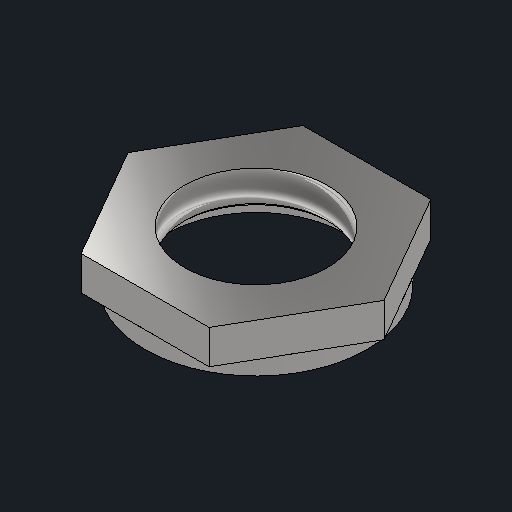
# Autodesk Inventor part: KN-00-02-03
Saved by Autodesk Inventor 2025.2 (Build 292293000, 293)
## iProperties
Created: 2025-04-12
Part Number: KN-00-02-03
Material: X5CrNi18-10
Document SubType Name: Modeling
Designer: Kacper Mik
Density: 8 g/cm^3
Appearance: Semi-Polished
Author: Kacper Mik
Autodesk Inventor part; units mm, degrees
ref_plane "YZ Plane" through (0, 0, 0) normal (1, 0, 0) x (0, 1, 0)
ref_plane "XZ Plane" through (0, 0, 0) normal (0, 1, 0) x (-1, 0, 0)
ref_plane "XY Plane" through (0, 0, 0) normal (0, 0, 1) x (1, 0, 0)
sketch "Sketch1" plane through (0, 0, 0) normal (0, 1, 0) x (-1, 0, 0)
  circle A0 centre (0, 0) radius 6.5
  line L0 (-3.7528, -6.5) -> (-7.5056, 0)
  line L1 (-7.5056, 0) -> (-3.7528, 6.5)
  line L2 (-3.7528, 6.5) -> (3.7528, 6.5)
  line L3 (3.7528, 6.5) -> (7.5056, 0)
  line L4 (7.5056, 0) -> (3.7528, -6.5)
  line L5 (3.7528, -6.5) -> (-3.7528, -6.5)
  point P0 (0, -6.5)
  point P1 (5.6292, -3.25)
  point P2 (-5.6292, -3.25)
  point P3 (5.6292, 3.25)
  point P4 (0, 6.5)
  point P5 (-5.6292, 3.25)
  dimension "d0" = 13
  constraints: 12 end point, 2 coincident, 1 midpoint, 16 other
extrude "Extrusion1" add sketch "Sketch1" along normal blind 2
sketch "Sketch3" plane through (0, 0, 0) normal (0, -1, 0) x (1, 0, 0)
  point P0 (0, 0)
  point P1 (0, 0)
  constraints: 1 coincident
hole "Hole2" at (0, 0, 0) direction (0, 1, 0) diameter 8.376 end through all thread size "M10x1.5" class "6H" standard "ISO Metric profile"
sketch "Sketch4" plane through (0, 0, 0) normal (0, -1, 0) x (1, 0, 0)
  circle A0 centre (0, 0) radius 5.25
  circle A1 centre (0, 0) radius 6.5
  dimension "d23" = 10.5
  dimension "d24" = 13
  constraints: 2 centre point, 2 coincident
  measures "d23" diameter of A0
  measures "d24" diameter of A1
extrude "Extrusion2" add sketch "Sketch4" along normal blind 1
chamfer "Chamfer3" distance 0.2 angle 45 1 edges at (0, 0, 4.188)
body "Solid1"
